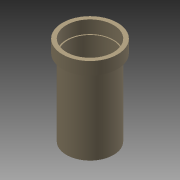
# Autodesk Inventor part: Outter Cup
Saved by Autodesk Inventor 2014 (Build 180170000, 170)
## iProperties
Created: 2014-06-10
Part Number: Outter Cup
Material: Generic
Document SubType Name: Modeling
Designer: Nabeel
Density: 1 g/cm^3
Appearance: Default
Author: Nabeel
Autodesk Inventor part; units mm, degrees
ref_plane "YZ Plane" through (0, 0, 0) normal (1, 0, 0) x (0, 1, 0)
ref_plane "XZ Plane" through (0, 0, 0) normal (0, 1, 0) x (-1, 0, 0)
ref_plane "XY Plane" through (0, 0, 0) normal (0, 0, 1) x (1, 0, 0)
sketch "Sketch1" plane through (0, 0, 0) normal (0, 0, 1) x (1, 0, 0)
  line L0 (-32.9, 0) -> (32.9, 0) projected
  line L1 (0, -32.9) -> (0, 32.9) projected
  circle A0 centre (0, 0) radius 23.5
  dimension "d0" = 47
  constraints: 1 centre point, 1 coincident
  measures "d0" diameter of A0
extrude "Extrusion1" add sketch "Sketch1" along normal blind 76.3
sketch "Sketch2" plane through (0, 0, 76.3) normal (0, 0, 1) x (1, 0, 0)
  circle A0 centre (0, 0) radius 23.5 projected
  circle A1 centre (0, 0) radius 27.5
  dimension "d3" = 55
  constraints: 1 centre point, 1 coincident
  measures "d3" diameter of A1
extrude "Extrusion2" add sketch "Sketch2" along normal blind 12.7
hole "Hole1" at (0.1504, 0.0752, 76.3) direction (0, 0, -1) diameter 45 depth 72
body "Solid1"
